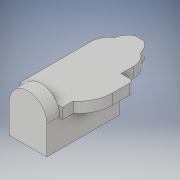
# Autodesk Inventor part: Space Envelope
Saved by Autodesk Inventor 2019 (Build 230136000, 136)
## iProperties
Created: 2021-02-11
Part Number: Space Envelope
Material: Generic
Document SubType Name: Modeling
Designer: Eric
Density: 1 g/cm^3
Appearance: Default
Author: Eric
Autodesk Inventor part; units mm, degrees
ref_plane "YZ Plane" through (0, 0, 0) normal (1, 0, 0) x (0, 1, 0)
ref_plane "XZ Plane" through (0, 0, 0) normal (0, 1, 0) x (-1, 0, 0)
ref_plane "XY Plane" through (0, 0, 0) normal (0, 0, 1) x (1, 0, 0)
sketch "Sketch1" plane through (0, 0, 0) normal (0, 0, 1) x (1, 0, 0)
  arc A0 (-16, 36.5624) -> (16, 36.5624) centre (0, 8.8496) ccw projected
  line L0 (-16, 36.5624) -> (0, 45.8) projected
  line L1 (0, 45.8) -> (16, 36.5624) projected
  line L2 (37.5, 8.8496) -> (37.5, -28.6504) projected
  arc A1 (37.5, 8.8496) -> (-37.5, 8.8496) centre (0, 8.8496) ccw projected
  line L3 (-37.5, -28.6504) -> (-37.5, 8.8496) projected
  line L4 (37.5, -28.6504) -> (-37.5, -28.6504) projected
  line L5 (-37.5, -28.6504) -> (37.5, -28.6504)
  line L6 (37.5, -28.6504) -> (37.5, -48.6504)
  line L7 (37.5, -48.6504) -> (-37.5, -48.6504)
  line L8 (-37.5, -48.6504) -> (-37.5, -28.6504)
  point P0 (0, 0)
  dimension "d0" = 20
  constraints: 8 end point, 3 collinear, 1 parallel
  measures "d0" distance of L5.end L6.end
ref_plane "Work Plane1" through (-37.4166, 11.3496, -26) normal (0, 0, -1) x (0, 1, 0)
extrude "Extrusion1" add sketch "Sketch1" against normal up to surface (26 mm away) contours L0 L1 A0 | L2 L4 L3 A1 | L6 L7 L8 L4
sketch "Sketch2" plane through (0, 8.8496, -26) normal (0, 0, -1) x (-1, 0, 0)
  line L0 (-37.5, -57.5) -> (-37.5, 0) projected
  line L1 (37.5, -57.5) -> (-37.5, -57.5) projected
  line L2 (37.5, 0) -> (37.5, -57.5) projected
  line L3 (-37.5, -3.5) -> (-28.6182, -3.5) projected
  line L4 (-37.5, -57.5) -> (37.5, -57.5)
  line L5 (37.5, -57.5) -> (37.5, -3.5)
  line L6 (37.5, -3.5) -> (-37.5, -3.5)
  line L7 (-37.5, -3.5) -> (-37.5, -57.5)
  point P0 (0, -8.8496)
  constraints: 8 end point, 4 collinear
ref_plane "Work Plane2" through (-37.5, -28.6504, -144) normal (0, 0, -1) x (0, 1, 0)
extrude "Extrusion2" add sketch "Sketch2" along normal up to surface (118 mm away)
sketch "Sketch3" plane through (-37.5, 5.3496, -26) normal (0, 1, 0) x (1, 0, 0)
  line L0 (75, 118) -> (0, 118) projected
  line L1 (0, 0) -> (0, 118) projected
  line L2 (75, 0) -> (0, 0) projected
  line L3 (75, 0) -> (75, 118) projected
  line L4 (80, 0) -> (-5, 0)
  line L5 (-5, 0) -> (-5, 142)
  line L6 (-5, 142) -> (80, 142)
  line L7 (80, 142) -> (80, 0)
  line L8 (37.5, 0) -> (37.5, 165)
  arc A0 (72.5, 142) -> (2.5, 142) centre (37.5, 142) ccw construction
  arc A1 (80, 142) -> (45, 177) centre (45, 142) ccw
  arc A2 (30, 177) -> (-5, 142) centre (30, 142) ccw
  line L9 (45, 177) -> (30, 177)
  line L10 (64.25, 165) -> (10.75, 165)
  arc A3 (45.75, 200) -> (10.75, 165) centre (45.75, 165) ccw
  line L11 (45.75, 165) -> (45.75, 200) construction
  line L12 (45.75, 165) -> (10.75, 165) construction
  arc A4 (64.25, 165) -> (29.25, 200) centre (29.25, 165) ccw
  line L13 (29.25, 165) -> (29.25, 200) construction
  line L14 (29.25, 165) -> (64.25, 165) construction
  line L15 (46, 195.7317) -> (29, 195.7317)
  line L16 (37.5, 109) -> (97.5, 109) construction
  circle A5 centre (97.5, 109) radius 7.5 construction
  arc A6 (80, 56.5596) -> (105, 109) centre (37.5, 109) ccw construction
  line L17 (105, 109) -> (105, 74)
  arc A7 (80, 21.5596) -> (105, 74) centre (37.5, 74) ccw
  line L18 (97.5, 116.5) -> (80, 116.5)
  arc A8 (105, 109) -> (97.5, 116.5) centre (97.5, 109) ccw
  point P0 (37.5, -26)
  point P1 (37.5, 118)
  point P2 (37.5, 142)
  dimension "d5" = 5
  dimension "d6" = 5
  dimension "d7" = 24
  dimension "d8" = 35
  dimension "d9" = 35
  dimension "d10" = 35
  dimension "d11" = 47
  dimension "d12" = 53.5
  dimension "d13" = 90
  dimension "d14" = 90
  dimension "d15" = 35
  dimension "d16" = 35
  dimension "d17" = 17
  dimension "d26" = 15
  dimension "d27" = 60
  dimension "d28" = 109
  dimension "d29" = 35
  constraints: 30 end point, 20 point on circle, 13 point on line, 9 centre point, 4 coincident, 4 midpoint, 4 parallel, 2 perpendicular, 2 tangent, 1 collinear, 1 equal radius
  measures "d5" distance between parallel lines of L5 L1
  measures "d6" distance between parallel lines of L3 L7
  measures "d7" distance between parallel lines of L6 L0
  measures "d8" radius of A0
  measures "d9" radius of A2
  measures "d10" radius of A1
  measures "d11" distance between parallel lines of L0 L10
  measures "d12" distance of L10.start L10.end
  measures "d13" angle of L11 L12
  measures "d14" angle of L14 L13
  measures "d15" radius of A4
  measures "d16" radius of A3
  measures "d17" distance of L15.start L15.end
  measures "d26" diameter of A5
  measures "d27" distance of L16.start L16.end
  measures "d28" distance of L8.start L16.start
  measures "d29" distance of L17.start L17.end
ref_plane "Work Plane3" through (-7.5, 26.4496, -42.5) normal (0, 1, 0) x (0, 0, 1)
extrude "Extrusion3" add sketch "Sketch3" along normal up to surface (21.1 mm away) contours L3 L2 L8 L0 | L0 L8 L6 L7 L4 L3 | L8 L2 L1 L0 | L0 L1 L4 L5 L6 L8 | L8 L10 A4 A1 L6 | L6 A2 A3 L10 L8 | L10 A3 A2 L9 A1 A4 | L7 L18 A8 L17 A7 | A3 L15 A4 A1 L9 A2
ref_plane "Work Plane4" through (12.5, 5.3496, -168) normal (-1, 0, 0) x (0, 0, 1)
ref_plane "Work Plane6" through (0, -1.1504, 0) normal (0, -1, 0) x (1, 0, 0)
ref_plane "Work Plane5" through (0, 46.3496, 0) normal (0, -1, 0) x (1, 0, 0)
ref_plane "Work Plane7" through (0, 0, -110.8659) normal (0, 0, 1) x (1, 0, 0)
equation "\"d9\" = d8"
equation "\"d10\" = d8"
equation "\"d15\" = d8"
equation "\"d16\" = d8"
body "Solid1"
